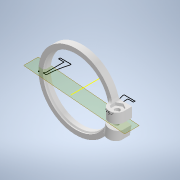
# Autodesk Inventor part: motor_frontalholder_retainerscrew
Saved by Autodesk Inventor 2020 (Build 240168000, 168)
## iProperties
Created: 2019-08-02
Part Number: motor_frontalholder_retainerscrew
Material: Generic
Document SubType Name: Modeling
Designer: erwin
Density: 1 g/cm^3
Appearance: Default
Author: erwin
Autodesk Inventor part; units mm, degrees
ref_plane "YZ Plane" through (0, 0, 0) normal (1, 0, 0) x (0, 1, 0)
ref_plane "XZ Plane" through (0, 0, 0) normal (0, 1, 0) x (-1, 0, 0)
ref_plane "XY Plane" through (0, 0, 0) normal (0, 0, 1) x (1, 0, 0)
sketch "Sketch1" plane through (0, 0, 0) normal (0, 1, 0) x (-1, 0, 0)
  line L0 (34, -12) -> (34, -13.5)
  line L1 (34, -13.5) -> (24, -13.5)
  line L2 (24, -13.5) -> (24, -12)
  arc A0 (24, -12) -> (27, 6) centre (-32.9953, 6.7492) ccw
  line L3 (27, 6) -> (29.8747, 6)
  line L4 (29.8747, 6) -> (29.8747, 5)
  line L5 (29.8747, 5) -> (29, 4)
  line L6 (29, 4) -> (29, -12)
  line L7 (29, -12) -> (34, -12)
  line L8 (-34, -13.5) -> (-34, -12)
  line L9 (-34, -12) -> (-29, -12)
  line L10 (-29, -12) -> (-29, 4)
  line L11 (-29, 4) -> (-29.8747, 5)
  line L12 (-29.8747, 5) -> (-29.8747, 6)
  line L13 (-29.8747, 6) -> (-27, 6)
  arc A1 (-27, 6) -> (-24, -12) centre (32.9953, 6.7492) ccw
  line L14 (-24, -12) -> (-24, -13.5)
  line L15 (-24, -13.5) -> (-34, -13.5)
  line L16 (-29, 0) -> (-34, 0)
  line L17 (-34, 0) -> (-34, 6)
  line L18 (-34, 6) -> (-29, 6)
  line L19 (-29, 6) -> (-29, 0)
  line L20 (0, -17.5498) -> (0, 10.7991) projected
  point P0 (0, 0)
  dimension "d0" = 5
  constraints: 40 end point, 8 vertical, 7 horizontal, 4 point on circle, 2 centre point, 2 parallel, 1 perpendicular, 1 point on line, 24 other
  measures "d0" distance of L17.end L18.end
revolve "Revolution1" add sketch "Sketch1" angle 360 about axis through (0, 0, -10) along (0, 0, 1) contours L16 L17 L18 L12 L11 L10
revolve "Revolution2" cut sketch "Sketch1" angle 10 about axis through (0, 0, -10) along (0, 0, -1) contours L16 L17 L18 L12 L11 L10
sketch "Sketch2" plane through (29, 0, 0) normal (0, -1, 0) x (1, 0, 0)
  circle A0 centre (9, 7) radius 3.5
  line L0 (5, 0) -> (-63, 0) projected
  circle A1 centre (9, 7) radius 7
  line L1 (15.9282, 6) -> (5, 6)
  line L2 (5, 6) -> (5, 0)
  line L3 (5, 0) -> (15.9282, 0)
  line L4 (15.9282, 0) -> (15.9282, 6)
  line L5 (5, 6) -> (-63, 6) projected
  line L6 (2.0718, 6) -> (2.0718, 0)
  point P0 (-29, 0)
  point P1 (4.4835, 0)
  point P2 (4.4835, 6)
  dimension "d3" = 7
  dimension "d4" = 7
  dimension "d5" = 4
  dimension "d6" = 14
  constraints: 10 end point, 2 centre point, 2 parallel, 2 point on circle, 2 point on line, 1 coincident, 1 horizontal, 1 perpendicular, 1 vertical
  measures "d3" diameter of A0
  measures "d4" distance from line of L0 A0.centre
  measures "d5" horizontal distance of A0.centre L0.start
  measures "d6" diameter of A1
extrude "Extrusion1" add sketch "Sketch2" against normal blind 8
sketch "Sketch4" plane through (33.4835, -5.904, 6) normal (0.1736482, 0.9848078, 0) x (0.9848078, -0.1736482, 0)
  line L0 (-5, 6) -> (0, 6) projected
  line L1 (-5, 2) -> (-5, 6) projected
  line L2 (-4.1253, 1) -> (-5, 2) projected
  line L3 (-4.1253, 0) -> (-4.1253, 1) projected
  line L4 (0, 0) -> (-4.1253, 0) projected
  line L5 (0, 6) -> (0, 0) projected
  line L6 (-4.1253, 0) -> (-4.1253, 1) projected
  point P0 (-34, 6)
  constraints: 1 coincident
ref_plane "Work Plane1" through (0, 0, 0) normal (-0.0871557, -0.9961947, 0) x (0, 0, -1)
mirror "Mirror1" about plane through (0, 0, 0) normal (-0.0871557, -0.9961947, 0) of "Extrusion1"
fillet "Fillet1" radius 2 2 edges at (29.9052, -9.3348, 6) (31.0718, 4, 6)
fillet "Fillet2" radius 3 6 edges at (28.2178, -13.099, 6) (30.1824, -13.4454, 6) (30.0638, 8, 6) (32.0586, 8, 6) (31.1542, -13.6167, 3) (33.0454, 8, 3)
sketch "Sketch8" plane through (0, 0, 0) normal (-0.0871557, -0.9961947, 0) x (0, 0, -1)
  ellipse E0 centre (-7, 37.8554) end of major axis (-14, 37.8554) minor radius 6.9734 (-6, 44.7572) -> (-7.7778, 30.9252) ccw projected
  circle A0 centre (-7, 37.8554) radius 2.25
  point P0 (0, 0)
  point P1 (-6, 30.9536)
  dimension "d28" = 4.5
  constraints: 1 centre point, 1 coincident, 1 other
  measures "d28" diameter of A0
extrude "Extrusion3" cut sketch "Sketch8" along normal through all both and the other way through all
sketch "Sketch9" plane through (29, 8, 0) normal (0, 1, 0) x (1, 0, 0)
  ellipse E0 centre (9.6999, -7) end of major axis (11.9585, -7) minor radius 2.25 projected
  line L0 (14.1999, -9.5981) -> (9.6999, -12.1962)
  line L1 (9.6999, -12.1962) -> (5.1999, -9.5981)
  line L2 (5.1999, -9.5981) -> (5.1999, -4.4019)
  line L3 (5.1999, -4.4019) -> (9.6999, -1.8038)
  line L4 (9.6999, -1.8038) -> (14.1999, -4.4019)
  line L5 (14.1999, -4.4019) -> (14.1999, -9.5981)
  line L6 (15.9282, -6) -> (15.9282, 0) projected
  point P0 (-29, 0)
  dimension "d31" = 9
  constraints: 12 end point, 1 coincident, 1 parallel, 13 other
  measures "d31" distance between parallel lines of L5 L2
extrude "Extrusion4" cut sketch "Sketch9" along normal mid plane 5 contours E0 | L0 L1 L2 L3 L4 L5
mirror "Mirror2" about plane through (0, 0, 0) normal (-0.0871557, -0.9961947, 0) of "Extrusion4"
move faces "Move1" translate (0, -1, 0) faces at (37.3094, 0, 1.5833)
move faces "Move2" translate (0.1736, 0.9848, 0) faces at (42.6414, -7.5188, 5.2919) (43.208, -7.6187, 1.2476) (30.2601, -5.3357, 1.6013) (30.0655, -5.3014, 6.0729)
body "Solid1"
